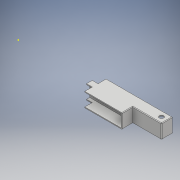
# Autodesk Inventor part: SoporteUV
Saved by Autodesk Inventor 2017 (Build 210142000, 142)
## iProperties
Created: 2021-01-04
Part Number: SoporteUV
Material: Generic
Document SubType Name: Modeling
Designer: USUARIO
Density: 1 g/cm^3
Appearance: Default
Author: USUARIO
Autodesk Inventor part; units mm, degrees
ref_plane "YZ Plane" through (0, 0, 0) normal (1, 0, 0) x (0, 1, 0)
ref_plane "XZ Plane" through (0, 0, 0) normal (0, 1, 0) x (-1, 0, 0)
ref_plane "XY Plane" through (0, 0, 0) normal (0, 0, 1) x (1, 0, 0)
sketch "Sketch1" plane through (0, 0, 0) normal (0, 1, 0) x (-1, 0, 0)
  line L0 (0, 0) -> (-500, 0)
  line L1 (-500, 0) -> (-500, -50)
  line L2 (-500, -50) -> (0, -50)
  line L3 (0, -50) -> (0, 0)
  dimension "d0" = 500
  dimension "d1" = 50
  constraints: 8 end point, 2 parallel, 1 horizontal, 1 perpendicular
  measures "d0" distance of L2.end L1.end
  measures "d1" distance of L1.end L0.end
extrude "Extrusion1" add sketch "Sketch1" along normal blind 2
sketch "Sketch2" plane through (0, 2, 0) normal (0, 1, 0) x (1, 0, 0)
  point P0 (0, 0)
sketch "Sketch3" plane through (0, 2, 0) normal (0, 1, 0) x (1, 0, 0)
  line L0 (0, 0) -> (500, 0)
  line L1 (500, 0) -> (500, 3)
  line L2 (500, 3) -> (0, 3)
  line L3 (0, 3) -> (0, 0)
  line L4 (0, 50) -> (0, 0) projected
  line L5 (0, 50) -> (500, 50)
  line L6 (500, 50) -> (500, 47)
  line L7 (500, 47) -> (0, 47)
  line L8 (0, 47) -> (0, 50)
  line L9 (500, 3) -> (497, 3)
  line L10 (497, 3) -> (497, 47)
  line L11 (497, 47) -> (500, 47)
  line L12 (500, 47) -> (500, 3)
  line L13 (0, 3) -> (3, 3)
  line L14 (3, 3) -> (3, 47)
  line L15 (3, 47) -> (0, 47)
  line L16 (0, 47) -> (0, 3)
  dimension "d4" = 500
  dimension "d5" = 3
  dimension "d6" = 500
  dimension "d7" = 3
  dimension "d8" = 3
  dimension "d9" = 44
  dimension "d10" = 3
  dimension "d11" = 44
  constraints: 32 end point, 8 parallel, 4 horizontal, 4 perpendicular
  measures "d4" distance of L2.end L1.end
  measures "d5" distance of L1.end L0.end
  measures "d6" distance of L6.end L7.end
  measures "d7" distance of L5.end L6.end
  measures "d8" distance of L10.end L11.end
  measures "d9" distance of L9.end L10.end
  measures "d10" distance of L15.end L14.end
  measures "d11" distance of L14.end L13.end
extrude "Extrusion2" add sketch "Sketch3" along normal blind 37 contours L3 L2 L1 L0 | L4 L7 L14 L2 | L2 L10 L7 L12 | L4 L5 L6 L7
sketch "Sketch4" plane through (0, 0, 0) normal (0, -1, 0) x (1, 0, 0)
  line L0 (0, 0) -> (400, 0)
  line L1 (400, 0) -> (400, -3)
  line L2 (400, -3) -> (0, -3)
  line L3 (0, -3) -> (0, 0)
  line L4 (500, -50) -> (0, -50) projected
  line L5 (0, -50) -> (400, -50)
  line L6 (400, -50) -> (400, -47)
  line L7 (400, -47) -> (0, -47)
  line L8 (0, -47) -> (0, -50)
  line L9 (0, -47) -> (3, -47)
  line L10 (3, -47) -> (3, -3)
  line L11 (3, -3) -> (0, -3)
  line L12 (0, -3) -> (0, -47)
  line L13 (400, -3) -> (397, -3)
  line L14 (397, -3) -> (397, -47)
  line L15 (397, -47) -> (400, -47)
  line L16 (400, -47) -> (400, -3)
  dimension "d14" = 400
  dimension "d15" = 3
  dimension "d16" = 400
  dimension "d17" = 3
  dimension "d18" = 3
  dimension "d19" = 44
  dimension "d20" = 3
  dimension "d21" = 44
  constraints: 32 end point, 8 parallel, 4 horizontal, 4 perpendicular
  measures "d14" distance of L1.end L2.end
  measures "d15" distance of L0.end L1.end
  measures "d16" distance of L7.end L6.end
  measures "d17" distance of L6.end L5.end
  measures "d18" distance of L11.end L10.end
  measures "d19" distance of L10.end L9.end
  measures "d20" distance of L15.end L14.end
  measures "d21" distance of L14.end L13.end
extrude "Extrusion3" add sketch "Sketch4" along normal blind 37 contours L0 L1 L2 L3 | L2 L10 L7 L12 | L16 L7 L14 L2 | L7 L6 L4 L8
fillet "Fillet1" radius 2 13 edges at (450, 0, 0) (450, 0, -50) (500, 0, -25) (500, 39, -25) (500, 19.5, 0) (500, 19.5, -50) (400, -18.5, 0) (400, -18.5, -50) (250, 39, 0) (250, 39, -50) (0, 1, 0) (0, 1, -50) (0, 39, -25)
fillet "Fillet2" radius 10 2 edges at (250, 2, -3) (250, 2, -47)
fillet "Fillet3" radius 10 2 edges at (250, 39, -3) (250, 39, -47)
sketch "Sketch5" plane through (2, 37, 0) normal (0, 0, 1) x (1, 0, 0)
  circle A0 centre (478.5, -17.5) radius 7.5
  line L0 (495, 2) -> (1, 2) projected
  line L1 (498, -35) -> (498, 0) projected
  point P0 (-2, -37)
  dimension "d27" = 15
  dimension "d28" = 19.5
  dimension "d29" = 19.5
  constraints: 1 centre point
  measures "d27" diameter of A0
  measures "d28" distance from line of L0 A0.centre
  measures "d29" distance from line of L1 A0.centre
extrude "Extrusion4" cut sketch "Sketch5" against normal blind 5
sketch "Sketch6" plane through (2, 37, 0) normal (0, 0, 1) x (1, 0, 0)
  line L0 (495, 2) -> (1, 2) projected
  line L1 (268, 2) -> (268, -28)
  line L2 (268, 2) -> (298, 2) construction
  line L3 (268, -28) -> (248, -28)
  line L4 (1, -25) -> (478.5, -25) projected
  line L5 (248, -28) -> (248, -48)
  line L6 (248, -48) -> (268, -48)
  line L7 (268, -48) -> (268, -74)
  line L8 (396, -74) -> (0, -74) projected
  line L9 (-2, 0) -> (-2, -74) projected
  point P0 (-2, -37)
  dimension "d32" = 30
  dimension "d33" = 270
  dimension "d34" = 20
  dimension "d35" = 90
  dimension "d36" = 20
  dimension "d37" = 20
  dimension "d38" = 250
  constraints: 12 end point, 4 point on line, 3 perpendicular, 1 horizontal, 1 parallel
  measures "d32" distance of L1.start L1.end
  measures "d34" distance of L1.end L3.end
  measures "d35" angle of L1 L3
  measures "d36" distance of L3.end L5.end
  measures "d37" distance of L5.end L6.end
  measures "d38" distance between parallel lines of L9 L5
split body "Split2" sketch "Sketch6" result one side removed curves L1 L3 L5 L6 L7 removed pieces at (85, -13.4206, -0.5)
body "Solid1"
